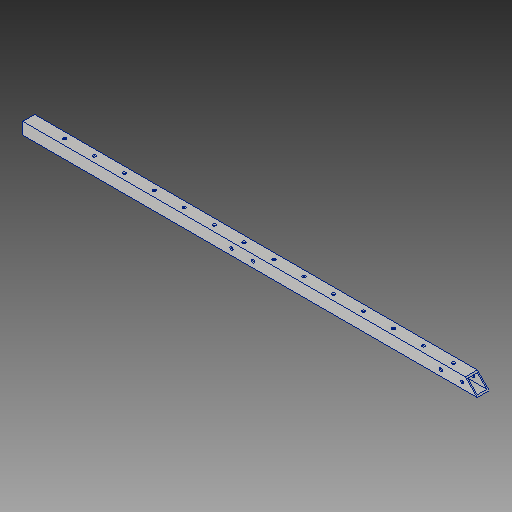
# Autodesk Inventor part: Secondary Extrusions
Saved by Autodesk Inventor 2019.4 (Build 234330000, 330)
## iProperties
Created: 2020-01-18
Part Number: Secondary Extrusions
Material: Aluminum 6061
Document SubType Name: Modeling
Designer: Mark
Mass: 286.981 g
Surface Area: 1078.81 cm^2
Volume: 106.289 cm^3
Density: 2.7 g/cm^3
Appearance: Aluminum - Flat
Author: Mark
Autodesk Inventor part; units mm, degrees
ref_plane "YZ Plane" through (0, 0, 0) normal (1, 0, 0) x (0, 1, 0)
ref_plane "XZ Plane" through (0, 0, 0) normal (0, 1, 0) x (-1, 0, 0)
ref_plane "XY Plane" through (0, 0, 0) normal (0, 0, 1) x (1, 0, 0)
sketch "Sketch1" plane through (0, 0, 0) normal (1, 0, 0) x (0, 1, 0)
  line L0 (-10, 10) -> (10, 10)
  line L1 (10, 10) -> (10, -10)
  line L2 (10, -10) -> (-10, -10)
  line L3 (-10, -10) -> (-10, 10)
  line L4 (-10, 10) -> (10, -10) construction
  line L5 (10, 10) -> (-10, -10) construction
  line L6 (-8, 8) -> (8, 8)
  line L7 (8, 8) -> (8, -8)
  line L8 (8, -8) -> (-8, -8)
  line L9 (-8, -8) -> (-8, 8)
  line L10 (-8, 8) -> (8, -8) construction
  line L11 (8, 8) -> (-8, -8) construction
  point P0 (0, 0)
  dimension "d0" = 20
  dimension "d1" = 20
  dimension "d2" = 16
  dimension "d3" = 16
  constraints: 24 end point, 4 midpoint, 4 parallel, 2 horizontal, 2 perpendicular
  measures "d0" distance of L1.end L2.end
  measures "d1" distance of L0.end L1.end
  measures "d2" distance of L7.end L8.end
  measures "d3" distance of L6.end L7.end
extrude "Extrusion1" add sketch "Sketch1" along normal blind 760
sketch "Sketch2" plane through (0, -10, -10) normal (0, 0, -1) x (-1, 0, 0)
  line L0 (0, 0) -> (-760, 0) projected
  line L1 (-760, 0) -> (-740, 20)
  line L2 (0, 20) -> (-760, 20) projected
  line L3 (-760, 0) -> (-760, 20) projected
  line L4 (0, 20) -> (-760, 20) projected
  line L5 (-20, 20) -> (0, 20)
  line L6 (0, 20) -> (0, 0)
  point P0 (0, 10)
  dimension "d6" = 20
  dimension "d9" = 20
  constraints: 6 end point, 2 point on line, 1 collinear
  measures "d6" distance from line of L3 L1.end
  measures "d9" distance of L2.start L5.start
extrude "Extrusion2" cut sketch "Sketch2" against normal blind 20 contours L3 L2 L1
sketch "Sketch3" plane through (760, -10, -10) normal (0, 0, -1) x (-1, 0, 0)
  circle A0 centre (25, 10) radius 2.75
  circle A1 centre (61, 10) radius 2.75
  line L0 (10, 10) -> (440, 10) construction
  line L1 (432, 18) -> (448, 2) projected
  line L2 (10, 10) -> (440, 10) construction
  line L3 (20, 20) -> (0, 0) projected
  circle A2 centre (375, 10) radius 2.75
  circle A3 centre (411, 10) radius 2.75
  dimension "d10" = 5.5
  dimension "d11" = 5.5
  dimension "d12" = 0
  dimension "d13" = 36
  dimension "d14" = 25
  dimension "d15" = 5.5
  dimension "d16" = 5.5
  dimension "d17" = 36
  dimension "d18" = 314
  constraints: 4 centre point, 4 end point, 4 point on line, 2 midpoint, 1 collinear, 1 horizontal
  measures "d10" diameter of A0
  measures "d11" diameter of A1
  measures "d12" distance between parallel lines of L0 L2
  measures "d13" distance of A0.centre A1.centre
  measures "d14" horizontal distance of L3.end A0.centre
  measures "d15" diameter of A2
  measures "d16" diameter of A3
  measures "d17" distance of A2.centre A3.centre
  measures "d18" distance of A1.centre A2.centre
extrude "Extrusion3" cut sketch "Sketch3" against normal blind 20
sketch "Sketch4" plane through (0, 10, 10) normal (0, 1, 0) x (1, 0, 0)
  circle A0 centre (60, 10) radius 2.75
  line L0 (0, 0) -> (0, 20) projected
  line L1 (0, 20) -> (740, 20) projected
  circle A1 centre (110, 10) radius 2.75
  circle A2 centre (160, 10) radius 2.75
  circle A3 centre (210, 10) radius 2.75
  circle A4 centre (260, 10) radius 2.75
  circle A5 centre (310, 10) radius 2.75
  circle A6 centre (360, 10) radius 2.75
  circle A7 centre (410, 10) radius 2.75
  circle A8 centre (460, 10) radius 2.75
  circle A9 centre (510, 10) radius 2.75
  circle A10 centre (560, 10) radius 2.75
  circle A11 centre (610, 10) radius 2.75
  circle A12 centre (660, 10) radius 2.75
  circle A13 centre (710, 10) radius 2.75
  circle A14 centre (760, 10) radius 2.75
  point P0 (0, 10)
  dimension "d21" = 5.5
  dimension "d22" = 60
  dimension "d23" = 10
  dimension "d26" = 50
  constraints: 15 centre point, 1 horizontal, 28 other
  measures "d21" diameter of A0
  measures "d22" distance from line of L0 A0.centre
  measures "d23" distance from line of L1 A0.centre
  measures "d26" distance of A0.centre A1.centre
extrude "Extrusion4" cut sketch "Sketch4" against normal blind 20 contours A0 | A1 | A2 | A3 | A4 | A5 | A6 | A7 | A8 | A9 | A10 | A11 | A12 | A13
body "Solid1"
